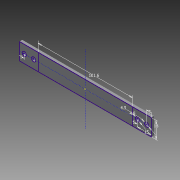
# Autodesk Inventor part: TopSliderBar
Saved by Autodesk Inventor 2014 SP1 (Build 180222100, 222)
## iProperties
Created: 2014-06-08
Part Number: TopSliderBar
Material: Generic
Document SubType Name: Modeling
Designer: Erin
Density: 1 g/cm^3
Appearance: Default
Author: Erin
Autodesk Inventor part; units mm, degrees
ref_plane "YZ Plane" through (0, 0, 0) normal (1, 0, 0) x (0, 1, 0)
ref_plane "XZ Plane" through (0, 0, 0) normal (0, 1, 0) x (-1, 0, 0)
ref_plane "XY Plane" through (0, 0, 0) normal (0, 0, 1) x (1, 0, 0)
sketch "Sketch1" plane through (0, 0, 0) normal (0, 1, 0) x (-1, 0, 0)
  line L0 (-70.8, 9) -> (0, 9)
  line L1 (70.8, 9) -> (70.8, -9)
  line L2 (70.8, -9) -> (0, -9)
  line L3 (-70.8, -9) -> (-70.8, 9)
  line L4 (-70.8, 0) -> (70.8, 0) construction
  circle A0 centre (-65.8, 0) radius 2.25
  circle A1 centre (-55.8, 0) radius 2.25
  line L5 (0, 9) -> (70.8, 9)
  line L6 (0, -9) -> (-70.8, -9)
  line L7 (-50.8, 9) -> (-50.8, -9)
  line L8 (0, 37.7423) -> (0, -37.3462) construction
  circle A2 centre (65.8, 0) radius 2.25
  circle A3 centre (55.8, 0) radius 2.25
  line L9 (50.8, 9) -> (50.8, -9)
  point P0 (0, 0)
  dimension "d1" = 18
  dimension "d2" = 4.5
  dimension "d3" = 4.5
  dimension "d4" = 5
  dimension "d5" = 15
  dimension "d17" = 5
  dimension "d18" = 101.6
  dimension "d19" = 5
  constraints: 20 end point, 6 parallel, 4 centre point, 4 perpendicular, 4 point on line, 4 symmetric about line, 2 horizontal, 2 midpoint, 1 horizontal alignment, 1 vertical, 1 vertical alignment, 2 other
  measures "d1" distance of L3.start L0.start
  measures "d2" diameter of A0
  measures "d3" diameter of A1
  measures "d4" distance from line of A0.centre L3
  measures "d5" distance from line of A1.centre L3
  measures "d17" distance from line of A1.centre L7
  measures "d18" distance between parallel lines of L9 L7
  measures "d19" distance from line of A2.centre L1
extrude "Extrusion1" add sketch "Sketch1" along normal blind 3
body "Solid1"
